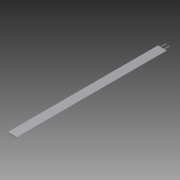
# Autodesk Inventor part: Ruler
Saved by Autodesk Inventor 2012 (Build 160160000, 160)
## iProperties
Created: 2013-07-07
Part Number: Ruler
Material: Default
Document SubType Name: Modeling
Designer: 1
Density: 1 g/cm^3
Author: 1
Autodesk Inventor part; units mm, degrees
ref_plane "YZ Plane" through (0, 0, 0) normal (1, 0, 0) x (0, 1, 0)
ref_plane "XZ Plane" through (0, 0, 0) normal (0, 1, 0) x (-1, 0, 0)
ref_plane "XY Plane" through (0, 0, 0) normal (0, 0, 1) x (1, 0, 0)
sketch "Sketch1" plane through (0, 0, 0) normal (0, 0, 1) x (1, 0, 0)
  arc A0 (112.5, 35.546) -> (107.5, 35.546) centre (110, 35.546) ccw projected
  arc A1 (107.5, 35.546) -> (112.5, 35.546) centre (110, 35.546) ccw projected
  arc A2 (87.5, 35.546) -> (92.5, 35.546) centre (90, 35.546) ccw projected
  arc A3 (92.5, 35.546) -> (87.5, 35.546) centre (90, 35.546) ccw projected
  line L0 (120, 31.7395) -> (120, 35.546) projected
  line L1 (120, 39.3526) -> (120, 35.546) projected
  line L2 (80, 39.3526) -> (80, 35.546) projected
  line L3 (80, 31.7395) -> (80, 35.546) projected
  line L4 (140, 34.046) -> (60, 34.046)
  line L5 (60, 34.046) -> (60, 37.046)
  line L6 (60, 37.046) -> (140, 37.046)
  line L7 (140, 37.046) -> (140, 34.046)
  line L8 (140, 37.046) -> (60, 34.046) construction
  line L9 (60, 37.046) -> (140, 34.046) construction
  line L10 (80, 35.546) -> (120, 35.546) construction
  point P0 (0, 0)
  point P1 (100, 35.546)
  dimension "d0" = 80
  dimension "d1" = 3
  constraints: 14 end point, 2 midpoint, 2 parallel, 2 perpendicular, 1 horizontal
  measures "d0" distance of L4.start L4.end
  measures "d1" distance of L6.end L4.start
extrude "Extrusion1" add sketch "Sketch1" along normal blind 850 contours A1 L4 A0 L6 | A0 L6 L1 L0 L4 A1 | A0 A1 L4 A2 A3 L6 | L6 L7 L4 L0 L1 | A3 A2 L4 L6 | A3 A2 L4 L3 L2 L6 | L2 L3 L4 L5 L6
sketch "Sketch2" plane through (0, 0, 0) normal (0, 0, -1) x (-1, 0, 0)
  arc A0 (-107.5, 35.546) -> (-112.5, 35.546) centre (-110, 35.546) ccw projected
  arc A1 (-112.5, 35.546) -> (-107.5, 35.546) centre (-110, 35.546) ccw projected
  arc A2 (-87.5, 35.546) -> (-92.5, 35.546) centre (-90, 35.546) ccw projected
  arc A3 (-92.5, 35.546) -> (-87.5, 35.546) centre (-90, 35.546) ccw projected
  circle A4 centre (-110, 35.546) radius 2.5
  circle A5 centre (-90, 35.546) radius 2.5
  point P0 (0, 0)
  constraints: 2 coincident, 2 horizontal alignment, 4 other
extrude "Extrusion2" add sketch "Sketch2" along normal blind 30.925 and the other way blind 7.5255
fillet "Fillet1" radius 0.9 6 edges at (110, 37.046, 7.5255) (108, 37.046, 3.7628) (92, 37.046, 3.7628) (90, 37.046, 7.5255) (88, 37.046, 3.7628) (112, 37.046, 3.7628)
fillet "Fillet2" radius 0.9 10 edges at (87.9368, 37.1148, 8.0804) (90, 38.046, 7.5255) (91.3052, 37.6783, 7.5663) (92.0632, 37.1148, 8.0804) (88.6948, 37.6783, 7.5662) (107.9368, 37.1148, 8.0804) (110, 38.046, 7.5255) (111.3052, 37.6783, 7.5663) (112.0632, 37.1148, 8.0804) (108.6948, 37.6783, 7.5662)
body "Solid1"
